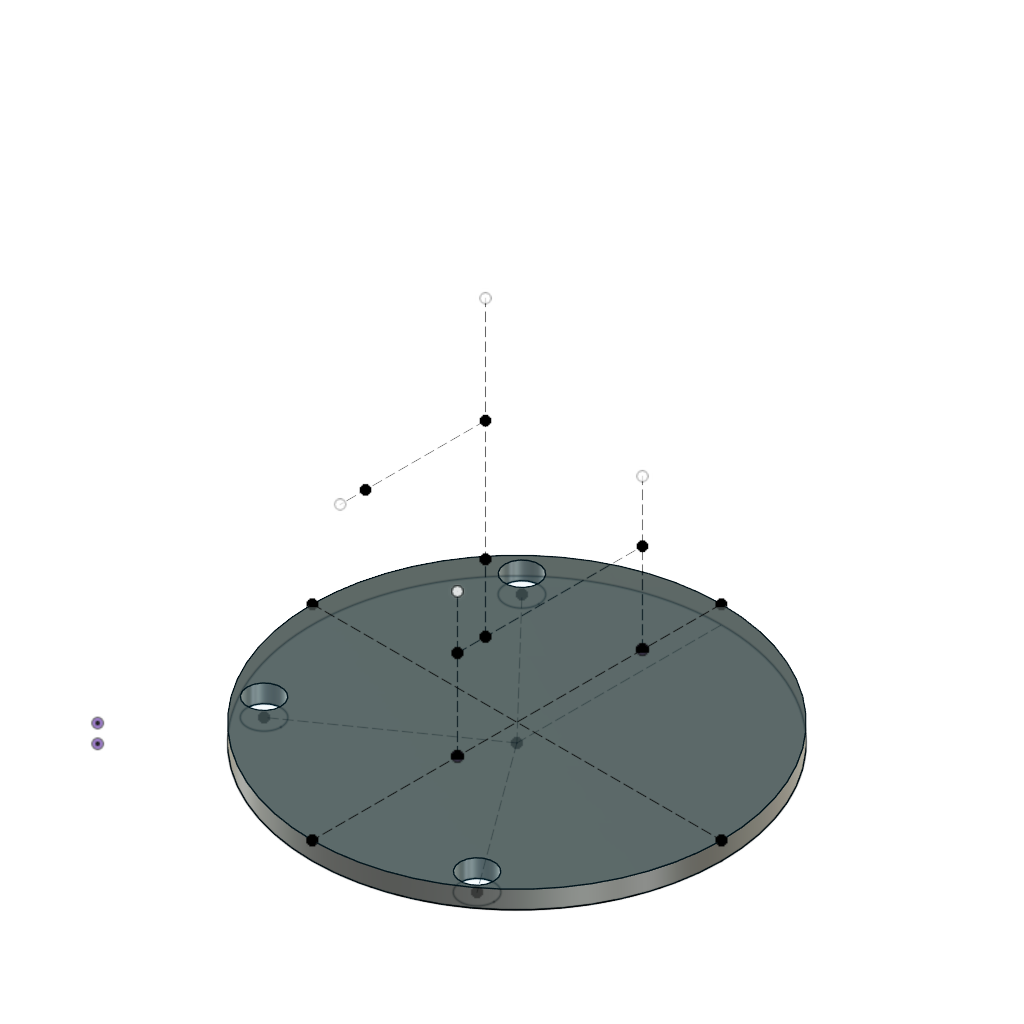
ZSB (Autodesk Fusion 360 archive; units mm, degrees)
design "Adapterplatine"
Autodesk Fusion 360 part; units mm, degrees
note: some values were not read from the file. Set by a fixed rule: which face or edge a step refers to.
sketch "Skizze1" plane through (0, 0, 0) normal (0, 0, 1) x (1, 0, 0)
  circle A0 centre (18.631, 18.76) radius 18.25
  circle A1 centre (7.381, 30.46) radius 1.5
  circle A2 centre (5.381, 9.46) radius 1.5
  circle A3 centre (28.381, 5.46) radius 1.5
  line L0 (18.631, 18.76) -> (7.381, 30.46) construction
  line L1 (18.631, 18.76) -> (5.381, 9.46) construction
  line L2 (18.631, 18.76) -> (28.381, 5.46) construction
  line L3 (18.631, 18.76) -> (18.631, 37.01) construction
  dimension "d1" = 36.5
  dimension "d4" = 18.631
  dimension "d5" = 18.76
  dimension "d6" = 3
  dimension "d7" = 7.381
  dimension "d8" = 30.46
  dimension "d9" = 9.46
  dimension "d10" = 5.381
  dimension "d11" = 5.46
  dimension "d12" = 28.381
  dimension "d24" = 43.877
  dimension "d25" = 125.065
  dimension "d26" = 143.756
  dimension "d27" = 16.2312
  dimension "d28" = 16.188
  dimension "d29" = 16.491
  constraint equal A1 A2
  constraint equal A1 A3
  constraint coincident A0.centre L0.start
  constraint coincident A1.centre L0.end
  constraint coincident A2.centre L1.end
  constraint coincident A3.centre L2.end
  constraint coincident A0 L3.end
  constraint vertical L3
  measures "d1" diameter of A0
  measures "d4" horizontal distance of origin A0.centre
  measures "d5" vertical distance of origin A0.centre
  measures "d6" diameter of A1
  measures "d7" horizontal distance of origin A1.centre
  measures "d8" vertical distance of origin A1.centre
  measures "d9" vertical distance of origin A2.centre
  measures "d10" horizontal distance of origin A2.centre
  measures "d11" vertical distance of origin A3.centre
  measures "d12" horizontal distance of origin A3.centre
  measures "d24" angle of L0 L3
  measures "d25" angle of L1 L3
  measures "d26" angle of L2 L3
  measures "d27" distance of A0.centre A1.centre
  measures "d28" distance of A0.centre A2.centre
  measures "d29" distance of A0.centre A3.centre
extrude "Extrusion1" add sketch "Skizze1" along normal blind 1.6
sketch "Skizze2" plane through (0, 0, 1.6) normal (0, 0, 1) x (-1, 0, 0)
  circle A0 centre (-5.381, -9.46) radius 1.5
  circle A1 centre (-7.381, -30.46) radius 1.5
  circle A2 centre (-28.381, -5.46) radius 1.5
  circle A3 centre (-18.631, -18.76) radius 18.25
  line L0 (-18.631, -37.01) -> (-18.631, -0.51) construction
  line L1 (-0.381, -18.76) -> (-36.881, -18.76) construction
  point P0 (-18.631, -29.96)
  point P1 (-18.631, -13.46)
  dimension "d13" = 13.46
  dimension "d15" = 29.96
  constraint coincident A3 L0.start
  constraint coincident A3 L0.end
  constraint vertical L0
  constraint coincident A3 L1.start
  constraint coincident A3 L1.end
  constraint horizontal L1
  constraint coincident A3.centre L1
  constraint coincident A3.centre L0
  constraint coincident L0 P1
  constraint coincident L0 P0
  measures "d13" vertical distance of origin P1
  measures "d15" vertical distance of origin P0
ref_plane "Arbeitsebene1" through (18.631, 0, 0) normal (1, 0, 0) x (0, 1, 0)
sketch "Skizze3" plane through (18.631, 0, 0) normal (1, 0, 0) x (0, 1, 0)
  line L0 (13.46, 1.6) -> (13.46, 14.3588) construction
  line L1 (29.96, 1.6) -> (29.96, 15) construction
  line L2 (13.46, 9.6) -> (29.96, 9.6) construction
  line L3 (15.96, 9.6) -> (15.96, 35.7478) construction
  line L4 (15.96, 26.3) -> (3, 26.3) construction
  point P0 (13.46, 1.6)
  point P1 (29.96, 1.6)
  point P2 (13.46, 9.6)
  point P3 (29.96, 9.6)
  point P4 (15.96, 9.6)
  point P5 (15.96, 15.6)
  point P6 (15.96, 26.3)
  point P7 (5.26, 26.3)
  dimension "d18" = 8
  dimension "d19" = 8
  dimension "d20" = 2.5
  dimension "d21" = 6
  dimension "d22" = 10.7
  dimension "d23" = 10.7
  constraint coincident P0 L0.start
  constraint vertical L0
  constraint coincident P1 L1.start
  constraint vertical L1
  constraint coincident L0 P2
  constraint coincident L1 P3
  constraint coincident P2 L2.start
  constraint coincident P3 L2.end
  constraint coincident L2 P4
  constraint coincident P4 L3.start
  constraint perpendicular L2 L3
  constraint coincident L3 P5
  constraint coincident L3 P6
  constraint coincident P6 L4.start
  constraint perpendicular L3 L4
  constraint coincident L4 P7
  measures "d18" distance of P0 P2
  measures "d19" distance of P1 P3
  measures "d20" distance of P2 P4
  measures "d21" distance of P4 P5
  measures "d22" distance of P5 P6
  measures "d23" distance of P6 P7
equation "d19 = d18"

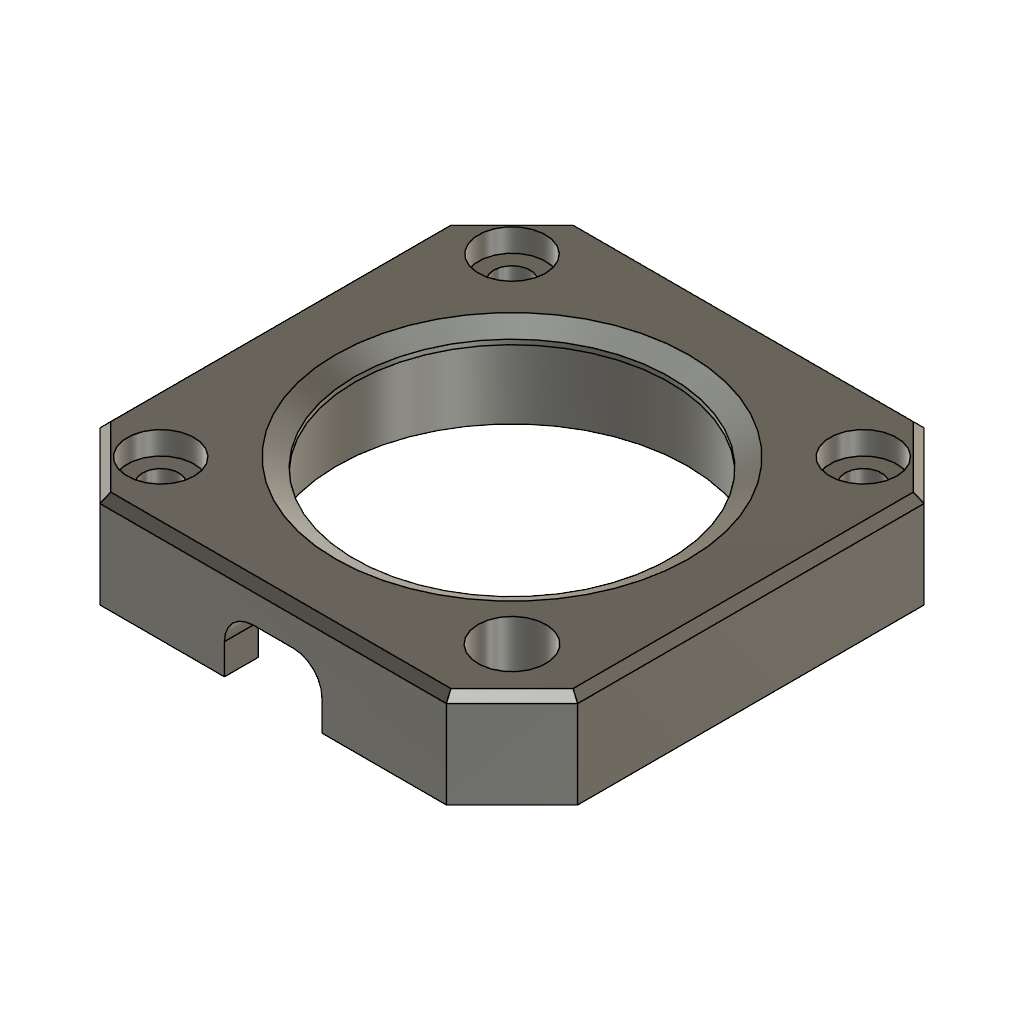
design "Frontplatte"
Autodesk Fusion 360 part; units mm, degrees
sketch "Skizze1" plane through (0, 0, 0) normal (0, 0, 1) x (1, 0, 0)
  line L0 (-50, 50) -> (0, 50)
  line L1 (0, 50) -> (0, 0)
  line L2 (0, 0) -> (-50, 0)
  line L3 (-50, 0) -> (-50, 50)
  line L4 (-50, 25) -> (0, 25) construction
  line L5 (-25, 50) -> (-25, 0) construction
  circle A0 centre (-25, 25) radius 16.5
  circle A1 centre (-8.0294, 8.0294) radius 3.55
  line L6 (-50, 50) -> (0, 0) construction
  line L7 (0, 50) -> (-50, 0) construction
  circle A2 centre (-43.3848, 43.3848) radius 1.9
  circle A3 centre (-6.6152, 43.3848) radius 1.9
  circle A4 centre (-43.3848, 6.6152) radius 1.9
  line L8 (-6.8665, 50) -> (0, 43.1335)
  line L9 (-50, 6.8665) -> (-43.1335, 0)
  line L10 (-43.1335, 50) -> (-50, 43.1335)
  line L11 (0, 6.8665) -> (-6.8665, 0)
  line L12 (-8.0294, 16.5147) -> (-16.5147, 8.0294) construction
  line L13 (-16.5147, 8.0294) -> (-8.0294, -0.4558) construction
  line L14 (-8.0294, -0.4558) -> (0.4558, 8.0294) construction
  line L15 (0.4558, 8.0294) -> (-8.0294, 16.5147) construction
  line L16 (-8.0294, 16.5147) -> (-8.0294, -0.4558) construction
  point P0 (-8.0294, 8.0294)
  point P1 (-8.0294, 8.0294)
  dimension "d3" = 33
  dimension "d4" = 7.1
  dimension "d6" = 3.8
  dimension "d7" = 26
  dimension "d8" = 26
  dimension "d9" = 26
  dimension "d42" = 50
  dimension "d43" = 50
  dimension "d44" = 61
  dimension "d45" = 61
  dimension "d46" = 12
  dimension "d47" = 12
  dimension "d54" = 6.5
  constraint horizontal L0
  constraint vertical L1
  constraint horizontal L2
  constraint vertical L3
  constraint coincident L1.end L2.start
  constraint midpoint L3 L4.start
  constraint midpoint L1 L4.end
  constraint midpoint L0 L5.start
  constraint midpoint L2 L5.end
  constraint midpoint L4 A0.centre
  constraint coincident L6 A2.centre
  constraint coincident L7 A3.centre
  constraint coincident L7 A4.centre
  constraint equal A2 A3
  constraint equal A2 A4
  constraint coincident L0 L8.start
  constraint coincident L1 L8.end
  constraint perpendicular L7 L8
  constraint coincident L3 L9.start
  constraint coincident L2 L9.end
  constraint perpendicular L7 L9
  constraint coincident L0 L10.start
  constraint coincident L3 L10.end
  constraint perpendicular L6 L10
  constraint coincident L1 L11.start
  constraint coincident L2 L11.end
  constraint symmetric L6 L8 L9
  constraint symmetric L7 L10 L11
  constraint coincident P1 P0
  constraint parallel L12 L14
  constraint vertical L16
  constraint perpendicular L12 L15
  constraint perpendicular L12 L13
  constraint midpoint L16 P1
  constraint coincident P1 L6
  measures "d3" diameter of A0
  measures "d4" diameter of A1
  measures "d6" diameter of A2
  measures "d7" distance of A0.centre A2.centre
  measures "d8" distance of A0.centre A3.centre
  measures "d9" distance of A0.centre A4.centre
  measures "d42" distance of L0.start L2.end
  measures "d43" distance of L0.start L0.end
  measures "d44" distance of L8 L9
  measures "d45" distance of L10 L11
  measures "d46" distance of L12.start L14.end
  measures "d47" distance of L12.start L12.end
  measures "d54" distance of P1 L11
extrude "Extrusion1" add sketch "Skizze1" along normal blind 3 contours L0 L1 L2 L3 L8 L9 L10 L11
chamfer "Fase1" distance 0.8 angle 45 8 edges at (-25, 0, 3) (-46.5668, 3.4332, 3) (-50, 25, 3) (-46.5668, 46.5668, 3) (-25, 50, 3) (-3.4332, 46.5668, 3) (0, 25, 3) (-3.4332, 3.4332, 3)
chamfer "Fase3" distance 2 distance2 1 1 edges at (-40.3834, 30.9667, 3) measured on face at (-24.589, 46.618, 3)
sketch "Skizze2" plane through (0, 0, 0) normal (0, 0, -1) x (1, 0, 0)
  circle A0 centre (-25, -25) radius 16.5
  circle A1 centre (-43.3848, -43.3848) radius 1.9
  circle A2 centre (-43.3848, -6.6152) radius 1.9
  circle A3 centre (-8.0294, -8.0294) radius 3.55
  circle A4 centre (-6.6152, -43.3848) radius 1.9
  line L0 (-50, -43.1335) -> (-43.1335, -50)
  line L1 (-43.1335, -50) -> (-6.8665, -50)
  line L2 (-6.8665, -50) -> (0, -43.1335)
  line L3 (0, -43.1335) -> (0, -6.8665)
  line L4 (0, -6.8665) -> (-6.8665, 0)
  line L5 (-6.8665, 0) -> (-43.1335, 0)
  line L6 (-43.1335, 0) -> (-50, -6.8665)
  line L7 (-50, -6.8665) -> (-50, -43.1335)
  circle A5 centre (-25, -25) radius 18.35
  line L8 (-14.75, -9.7796) -> (-17.9, -3.55)
  line L9 (-17.9, -3.55) -> (-32.1, -3.55)
  line L10 (-32.1, -3.55) -> (-35.25, -9.7796)
  line L11 (-25, -25) -> (-25, 4.0219) construction
  dimension "d18" = 36.7
  dimension "d19" = 21.45
  dimension "d20" = 20.5
  dimension "d21" = 14.2
  constraint concentric A0 A5
  constraint coincident A5 L8.start
  constraint horizontal L9
  constraint coincident A5 L10.end
  constraint coincident A0.centre A5.centre
  constraint vertical L11
  constraint symmetric L8.end L9.end L11
  constraint symmetric L8.start L10.end L11
  measures "d18" diameter of A5
  measures "d19" distance of A0.centre L9
  measures "d20" distance of L8.start L10.end
  measures "d21" distance of L8.end L9.end
extrude "Extrusion2" cut sketch "Skizze2" against normal blind 1.5 contours A5 | A5 L8 L9 L10
sketch "Skizze3" plane through (0, 0, 0) normal (0, -1, 0) x (1, 0, 0)
  line L0 (-6.8665, 2.2) -> (-43.1335, 2.2)
  line L1 (-43.1335, 2.2) -> (-43.1335, 0)
  line L2 (-43.1335, 0) -> (-6.8665, 0)
  line L3 (-6.8665, 0) -> (-6.8665, 2.2)
  line L4 (-41.5, 1.5) -> (-8.5, 1.5)
  line L5 (-41.5, 2) -> (-8.5, 2)
  line L6 (-25, 1.5) -> (-25, -10) construction
  line L7 (-22.9, -6.8) -> (-27.1, -6.8)
  line L8 (-22.9, -0.8) -> (-27.1, -0.8)
  arc A0 (-27.1, -0.8) -> (-27.1, -6.8) centre (-27.1, -3.8) ccw
  arc A1 (-22.9, -6.8) -> (-22.9, -0.8) centre (-22.9, -3.8) ccw
  line L9 (-19.9, -3.8) -> (-30.1, -3.8) construction
  line L10 (-25, -5.5) -> (-25, -2.1) construction
  line L11 (-22.9, -6.8) -> (-19.9, -6.8)
  line L12 (-19.9, -6.8) -> (-19.9, -3.8)
  line L13 (-27.1, -6.8) -> (-30.1, -6.8)
  line L14 (-30.1, -6.8) -> (-30.1, -3.8)
  line L15 (-30.1, -6.8) -> (-19.9, -6.8)
  line L16 (-19.9, -6.8) -> (-19.9, -8.8)
  line L17 (-19.9, -8.8) -> (-30.1, -8.8)
  line L18 (-30.1, -8.8) -> (-30.1, -6.8)
  point P0 (-25, -2.1)
  point P1 (-25, -5.5)
  point P2 (-25, -3.8)
  point P3 (-25, -3.8)
  dimension "d24" = 3.6
  dimension "d25" = 7
  dimension "d27" = 6
  dimension "d31" = 10.2
  dimension "d53" = 2
  constraint midpoint L4 L6.start
  constraint perpendicular L2 L6
  constraint coincident L6 P0
  constraint coincident L6 P1
  constraint horizontal L7
  constraint horizontal L8
  constraint tangent L7 A1
  constraint tangent L7 A0
  constraint tangent L8 A0
  constraint tangent L8 A1
  constraint symmetric L6 A1.centre A0.centre
  constraint coincident A1 L9.start
  constraint midpoint A0 L9.end
  constraint horizontal L9
  constraint coincident P1 L10.start
  constraint coincident P0 L10.end
  constraint midpoint L10 P3
  constraint midpoint L9 P3
  constraint coincident P3 P2
  constraint parallel L7 L11
  constraint perpendicular L7 L12
  constraint horizontal L13
  constraint perpendicular L13 L14
  constraint coincident L7.start A1.start
  constraint coincident L7.end A0.end
  constraint coincident L9.start L12.end
  constraint coincident L9.end L14.end
  constraint horizontal L15
  constraint vertical L16
  constraint horizontal L17
  constraint vertical L18
  constraint coincident L11.end L12.start
  measures "d24" distance of L6.start P0
  measures "d25" distance of L6.start P1
  measures "d27" distance of L7 L8
  measures "d31" distance of L9.start L9.end
  measures "d53" distance of L13.end L17.end
extrude "Extrusion3" add 1 faces at (-47.7677, 25.4366, 0) along direction (0, 0, -1) blind 7
extrude "Extrusion4" cut sketch "Skizze3" against normal up to surface (3.55 mm away) contours L7 L11 L13 L15 L16 L17 L18 | L7 L8 A0 A1 L15 | A1 L11 L12 L15 | A0 L13 L14 L15
sketch "Skizze4" plane through (0, 0, -7) normal (0, 0, -1) x (1, 0, 0)
  circle A0 centre (-43.3848, -43.3848) radius 1.9
  circle A1 centre (-6.6152, -43.3848) radius 1.9
  arc A2 (-35.25, -9.7796) -> (-14.75, -9.7796) centre (-25, -25) ccw
  arc A3 (-35.25, -9.7796) -> (-14.75, -9.7796) centre (-25, -25) ccw
  circle A4 centre (-8.0294, -8.0294) radius 3.55
  circle A5 centre (-8.0294, -8.0294) radius 3.55
  circle A6 centre (-43.3848, -6.6152) radius 1.9
  circle A7 centre (-8.0294, -8.0294) radius 3.5
  circle A8 centre (-8.0294, -8.0294) radius 5
  circle A9 centre (-6.6152, -43.3848) radius 1.1
  circle A10 centre (-6.6152, -43.3848) radius 3
  circle A11 centre (-43.3848, -43.3848) radius 1.1
  circle A12 centre (-43.3848, -43.3848) radius 3
  circle A13 centre (-43.3848, -6.6152) radius 1.1
  circle A14 centre (-43.3848, -6.6152) radius 3
  circle A15 centre (-43.3848, -43.3848) radius 1.9
  circle A16 centre (-6.6152, -43.3848) radius 1.9
  circle A17 centre (-43.3848, -6.6152) radius 1.9
  dimension "d49" = 6
  dimension "d50" = 10
  constraint concentric A4 A7
  constraint concentric A7 A8
  constraint concentric A1 A9
  constraint concentric A1 A10
  constraint concentric A0 A11
  constraint concentric A0 A12
  constraint concentric A6 A13
  constraint concentric A6 A14
  constraint equal A12 A14
  constraint equal A10 A12
  measures "d49" diameter of A14
  measures "d50" diameter of A8
extrude "Extrusion5" cut sketch "Skizze4" against normal blind 4 contours A10 | A12 | A14
extrude "Extrusion6" cut sketch "Skizze4" against normal blind 3 contours A8
sketch "Skizze5" plane through (0, 0, 3) normal (0, 0, 1) x (-1, 0, 0)
  line L0 (7.1979, -49.2) -> (42.8021, -49.2)
  line L1 (42.8021, -49.2) -> (49.2, -42.8021)
  line L2 (49.2, -42.8021) -> (49.2, -7.1979)
  line L3 (49.2, -7.1979) -> (42.8021, -0.8)
  line L4 (42.8021, -0.8) -> (7.1979, -0.8)
  line L5 (7.1979, -0.8) -> (0.8, -7.1979)
  line L6 (0.8, -7.1979) -> (0.8, -42.8021)
  line L7 (0.8, -42.8021) -> (7.1979, -49.2)
  circle A0 centre (43.3848, -43.3848) radius 1.9
  circle A1 centre (43.3848, -6.6152) radius 1.9
  circle A2 centre (6.6152, -43.3848) radius 1.9
  circle A3 centre (8.0294, -8.0294) radius 3.55
  circle A4 centre (25, -25) radius 18.5
  circle A5 centre (6.6152, -43.3848) radius 1.9
  circle A6 centre (6.6152, -43.3848) radius 1.9
  circle A7 centre (43.3848, -43.3848) radius 1.9
  circle A8 centre (43.3848, -43.3848) radius 1.9
  circle A9 centre (43.3848, -6.6152) radius 1.9
  circle A10 centre (43.3848, -6.6152) radius 1.9
  circle A11 centre (43.3848, -43.3848) radius 3.5
  circle A12 centre (43.3848, -6.6152) radius 3.5
  circle A13 centre (6.6152, -43.3848) radius 3.5
  dimension "d55" = 7
  constraint concentric A7 A11
  constraint concentric A9 A12
  constraint concentric A5 A13
  constraint equal A11 A13
  constraint equal A11 A12
  measures "d55" diameter of A11
extrude "Extrusion7" cut sketch "Skizze5" against normal blind 2.4 contours A11 | A12 | A13
sketch "Skizze6" plane through (0, 0, -7) normal (0, 0, -1) x (1, 0, 0)
  circle A0 centre (-8.0294, -8.0294) radius 5
  line L0 (-30.1, -3.55) -> (-30.1, 0)
  line L1 (-30.1, 0) -> (-43.1335, 0)
  line L2 (-43.1335, 0) -> (-50, -6.8665)
  line L3 (-50, -6.8665) -> (-50, -43.1335)
  line L4 (-50, -43.1335) -> (-43.1335, -50)
  line L5 (-43.1335, -50) -> (-6.8665, -50)
  line L6 (-6.8665, -50) -> (0, -43.1335)
  line L7 (0, -43.1335) -> (0, -6.8665)
  line L8 (0, -6.8665) -> (-6.8665, 0)
  line L9 (-6.8665, 0) -> (-19.9, 0)
  line L10 (-19.9, 0) -> (-19.9, -3.55)
  line L11 (-19.9, -3.55) -> (-17.9, -3.55)
  line L12 (-17.9, -3.55) -> (-14.75, -9.7796)
  arc A1 (-35.25, -9.7796) -> (-14.75, -9.7796) centre (-25, -25) ccw
  line L13 (-35.25, -9.7796) -> (-32.1, -3.55)
  line L14 (-32.1, -3.55) -> (-30.1, -3.55)
  circle A2 centre (-6.6152, -43.3848) radius 3
  circle A3 centre (-43.3848, -43.3848) radius 3
  circle A4 centre (-43.3848, -6.6152) radius 3
  circle A5 centre (-6.6152, -43.3848) radius 3
  circle A6 centre (-43.3848, -43.3848) radius 3
  circle A7 centre (-43.3848, -6.6152) radius 3
  circle A8 centre (-8.0294, -8.0294) radius 5
  circle A9 centre (-25, -25) radius 19.5
  dimension "d58" = 39
  constraint concentric A2 A5
  constraint concentric A3 A6
  constraint concentric A4 A7
  constraint concentric A0 A8
  constraint concentric A1 A9
  measures "d58" diameter of A9
equation "d8 = d7"
equation "d9 = d7"
equation "d54 = 6.85 mm - 0.35 mm"

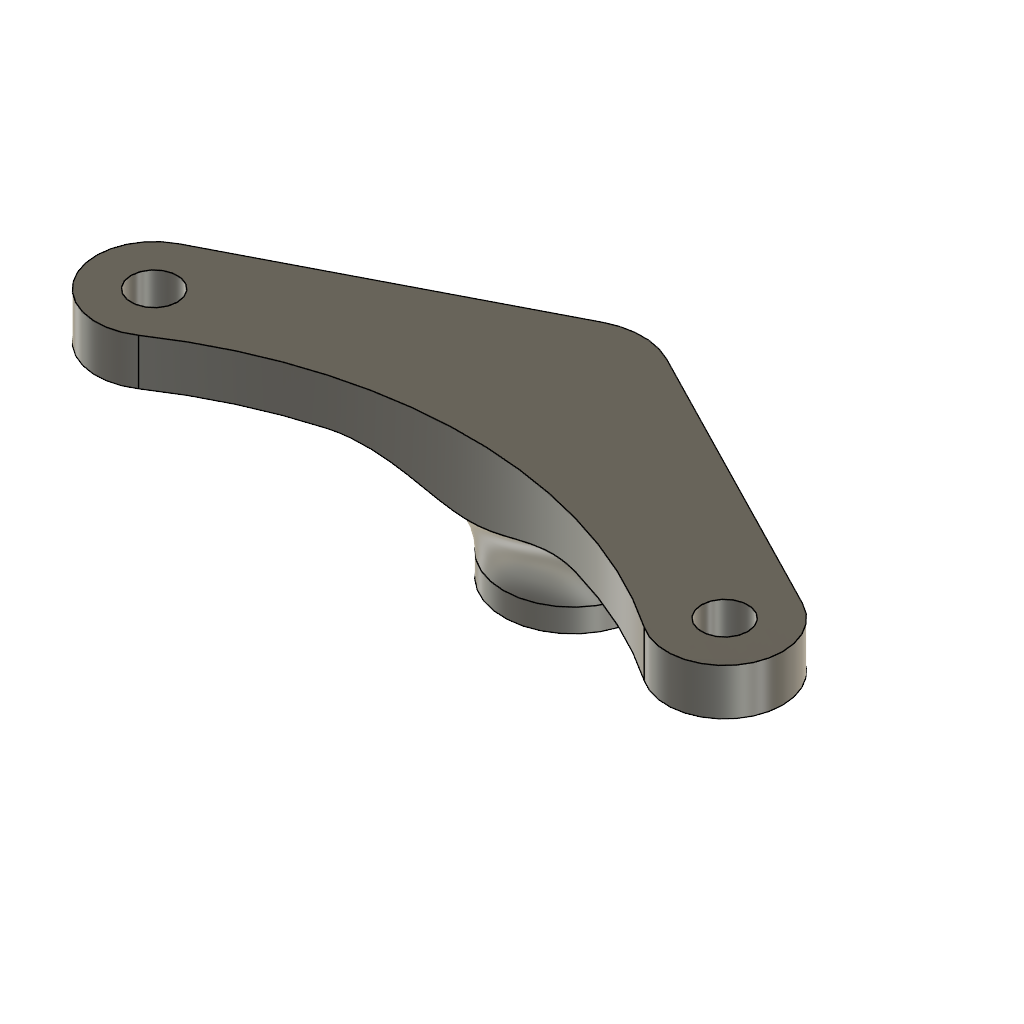
design "Haltebrücke"
Autodesk Fusion 360 part; units mm, degrees
sketch "Skizze1" plane through (0, 0, 0) normal (0, 0, 1) x (1, 0, 0)
  circle A0 centre (0, 0) radius 22 construction
  circle A1 centre (-12.3022, 18.2388) radius 1
  circle A2 centre (12.3022, 18.2388) radius 1
  line L0 (0, 0) -> (0, 38.9459) construction
  line L1 (0, 0) -> (-12.3022, 18.2388) construction
  line L2 (0, 0) -> (12.3022, 18.2388) construction
  circle A3 centre (-12.3022, 18.2388) radius 2.5
  circle A4 centre (12.3022, 18.2388) radius 2.5
  circle A5 centre (0, 24) radius 3
  line L3 (-1.3714, 26.6682) -> (-13.4451, 20.4623)
  line L4 (13.4451, 20.4623) -> (1.3714, 26.6682)
  arc A6 (10.9043, 16.1662) -> (-10.9043, 16.1662) centre (0, 0) ccw construction
  arc A7 (10.9043, 16.1662) -> (-10.9043, 16.1662) centre (0, 0) ccw
  point P0 (0, 24)
  dimension "d3" = 2
  dimension "d5" = 68
  dimension "d6" = 5
  dimension "d9" = 24
  dimension "d10" = 6
  dimension "d15" = 44
  dimension "d16" = 19.5
  constraint coincident A0.centre L0.start
  constraint coincident A0 A1.centre
  constraint coincident A0 A2.centre
  constraint vertical L0
  constraint coincident A1.centre L1.end
  constraint coincident A2.centre L2.end
  constraint symmetric A1.centre A2.centre L0
  constraint concentric A1 A3
  constraint concentric A2 A4
  constraint equal A1 A2
  constraint equal A3 A4
  constraint coincident L0 P0
  constraint coincident P0 A5.centre
  constraint coincident A5 L3.start
  constraint coincident A3 L3.end
  constraint coincident A4 L4.start
  constraint coincident A5 L4.end
  constraint tangent A5 L4
  constraint tangent A5 L3
  constraint tangent A3 L3
  constraint tangent A4 L4
  constraint concentric A0 A7
  constraint coincident L1 A6.end
  constraint coincident L2 A6.start
  constraint tangent A3 A6
  measures "d3" diameter of A1
  measures "d5" angle of L1 L2
  measures "d6" diameter of A3
  measures "d9" distance of A0.centre P0
  measures "d10" diameter of A5
  measures "d15" diameter of A0
  measures "d16" radius of A7
extrude "Extrusion1" add sketch "Skizze1" along normal blind 2
extrude "Extrusion2" add sketch "Skizze1" against normal blind 5.5 contours A5
fillet "Abrundung1" radius 4.5 1 edges at (0, 21, 0)

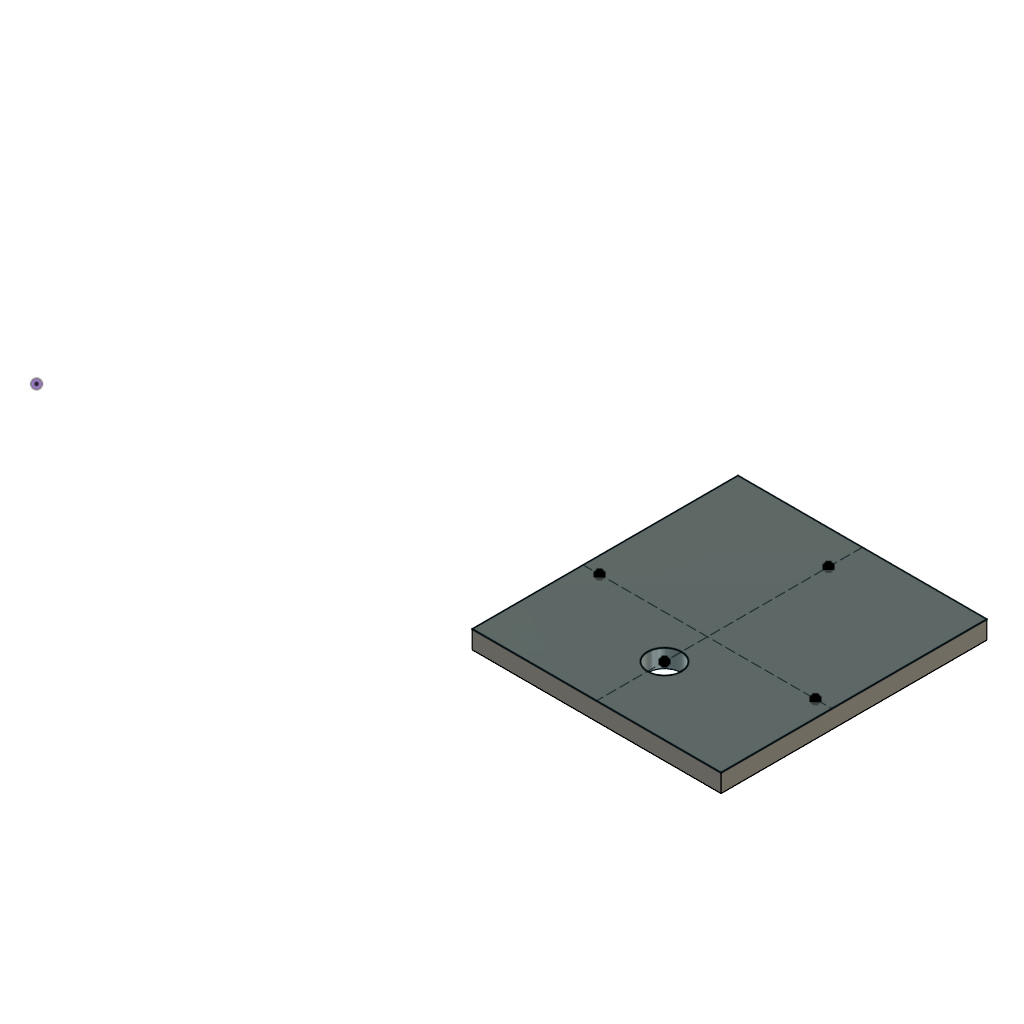
design "Adapter"
Autodesk Fusion 360 part; units mm, degrees
sketch "Skizze1" plane through (0, 0, 0) normal (0, 0, 1) x (1, 0, 0)
  line L0 (38, 23.99) -> (60, 23.99)
  line L1 (60, 23.99) -> (60, 0.49)
  line L2 (60, 0.49) -> (38, 0.49)
  line L3 (38, 0.49) -> (38, 23.99)
  circle A0 centre (49, 6.49) radius 1.5
  line L4 (49, 23.99) -> (49, 0.49) construction
  line L5 (38, 10.29) -> (60, 10.29) construction
  point P0 (39.46, 10.29)
  point P1 (58.54, 10.29)
  point P2 (49, 20.99)
  dimension "d1" = 38
  dimension "d2" = 60
  dimension "d3" = 0.49
  dimension "d4" = 23.99
  dimension "d5" = 3
  dimension "d7" = 6.49
  dimension "d8" = 10.29
  dimension "d9" = 39.46
  dimension "d10" = 58.54
  dimension "d11" = 20.99
  constraint horizontal L0
  constraint vertical L1
  constraint horizontal L2
  constraint vertical L3
  constraint midpoint L0 L4.start
  constraint midpoint L2 L4.end
  constraint coincident L3 L5.start
  constraint coincident L1 L5.end
  constraint perpendicular L1 L5
  constraint coincident A0.centre L4
  constraint coincident L5 P0
  constraint coincident L5 P1
  constraint coincident L4 P2
  measures "d1" horizontal distance of origin L2.end
  measures "d2" horizontal distance of origin L1.end
  measures "d3" vertical distance of origin L2.end
  measures "d4" vertical distance of origin L0.start
  measures "d5" diameter of A0
  measures "d7" vertical distance of origin A0.centre
  measures "d8" vertical distance of origin L5.start
  measures "d9" horizontal distance of origin P0
  measures "d10" horizontal distance of origin P1
  measures "d11" vertical distance of origin P2
extrude "Extrusion1" add sketch "Skizze1" against normal blind 1.6

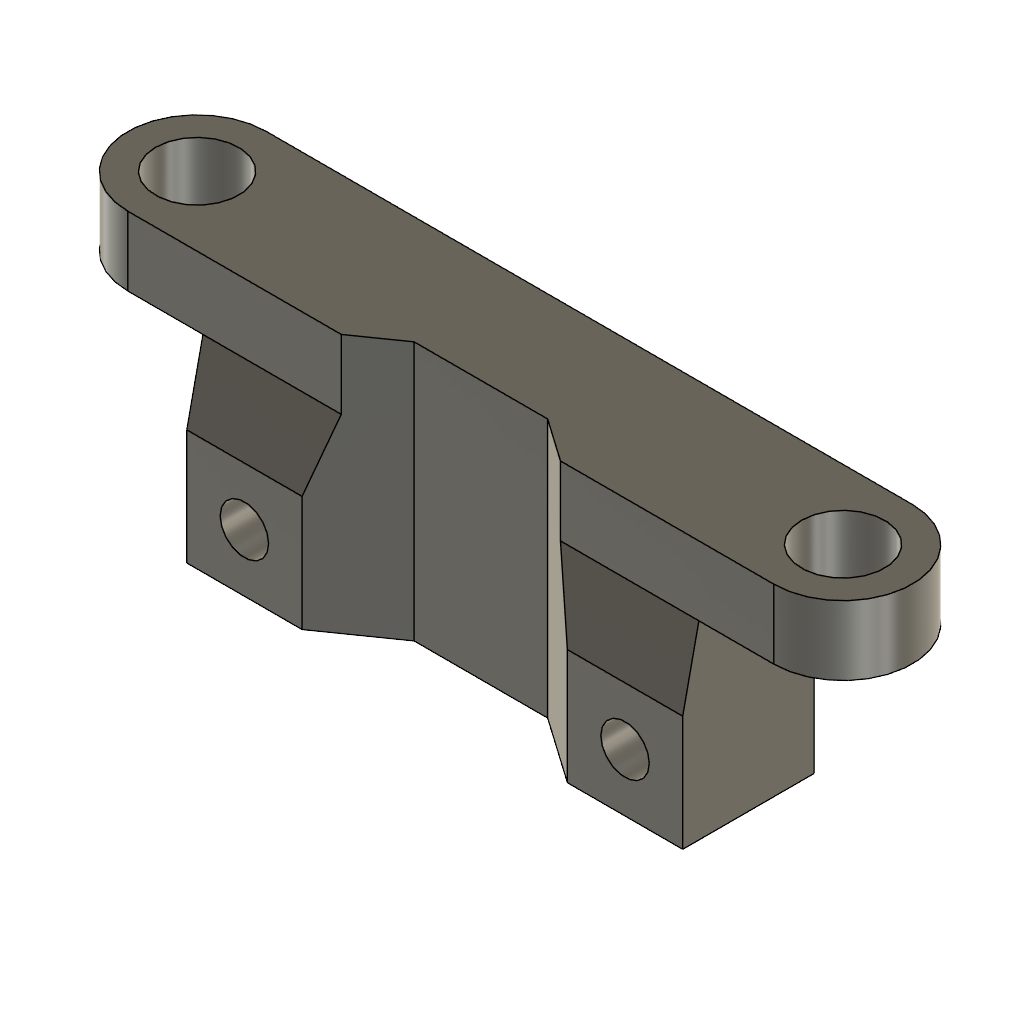
design "USB Halter"
Autodesk Fusion 360 part; units mm, degrees
sketch "Skizze1" plane through (0, 0, 0) normal (0, 0, 1) x (1, 0, 0)
  circle A0 centre (0, 0) radius 1.8
  circle A1 centre (-28, 0) radius 1.8
  line L0 (-28, 0) -> (0, 0) construction
  line L1 (-28, 3) -> (0, 3)
  line L2 (-28, -3) -> (0, -3)
  arc A2 (-28, 3) -> (-28, -3) centre (-28, 0) ccw
  arc A3 (0, -3) -> (0, 3) centre (0, 0) ccw
  dimension "d1" = 3.6
  dimension "d2" = 28
  dimension "d3" = 6
  constraint coincident A0.centre L0.end
  constraint coincident A1.centre L0.start
  constraint horizontal L0
  constraint equal A0 A1
  constraint concentric A1 A2
  constraint equal A2 A3
  constraint horizontal L1
  constraint parallel L0 L2
  constraint tangent L1 A3
  constraint tangent L2 A3
  measures "d1" diameter of A1
  measures "d2" distance of A0.centre A1.centre
  measures "d3" diameter of A2
extrude "Extrusion1" add sketch "Skizze1" along normal blind 3
sketch "Skizze2" plane through (0, 0, 0) normal (0, 0, 1) x (-1, 0, 0)
  circle A0 centre (0, 0) radius 1.8
  circle A1 centre (28, 0) radius 1.8
  arc A2 (28, -3) -> (28, 3) centre (28, 0) ccw
  line L0 (28, 3) -> (0, 3)
  arc A3 (0, 3) -> (0, -3) centre (0, 0) ccw
  line L1 (0, -3) -> (28, -3)
  line L2 (24.75, -3) -> (3.25, -3)
  line L3 (3.25, -3) -> (3.25, 3.7)
  line L4 (3.25, 3.7) -> (24.75, 3.7)
  line L5 (24.75, 3.7) -> (24.75, -3)
  circle A4 centre (0, 0) radius 1.8
  circle A5 centre (28, 0) radius 1.8
  arc A6 (28, -3) -> (28, 3) centre (28, 0) ccw
  line L6 (28, -3) -> (0, -3)
  arc A7 (0, 3) -> (0, -3) centre (0, 0) ccw
  line L7 (0, 3) -> (28, 3)
  line L8 (28, 0) -> (0, 0) construction
  line L9 (14, 0) -> (14, 18.5057) construction
  dimension "d9" = 0.7
  dimension "d10" = 21.5
  constraint horizontal L2
  constraint vertical L3
  constraint horizontal L4
  constraint vertical L5
  constraint coincident L1 L2.start
  constraint coincident A1.centre A2.centre
  constraint coincident A0.centre A3.centre
  constraint midpoint L8 L9.start
  constraint perpendicular L8 L9
  constraint symmetric L3 L5 L9
  measures "d9" distance of L0 L4
  measures "d10" distance of L3.end L4.end
extrude "Extrusion2" add sketch "Skizze2" against normal blind 8.23 contours L0 L1 L2 L3 L5 L6 L7 | L0 L3 L4 L5 L7
sketch "Skizze3" plane through (0, 3, 0) normal (0, 1, 0) x (-1, 0, 0)
  line L0 (24.75, 0) -> (28, 0)
  line L1 (28, 0) -> (28, 3)
  line L2 (28, 3) -> (0, 3)
  line L3 (0, 3) -> (0, 0)
  line L4 (0, 0) -> (3.25, 0)
  line L5 (3.25, 0) -> (3.25, -8.23)
  line L6 (3.25, -8.23) -> (24.75, -8.23)
  line L7 (24.75, -8.23) -> (24.75, 0)
  circle A0 centre (22.25, -5.73) radius 1.05
  circle A1 centre (5.75, -5.73) radius 1.05
  line L8 (24.75, -5.73) -> (3.25, -5.73) construction
  dimension "d11" = 2.1
  dimension "d13" = 2.5
  dimension "d14" = 2.5
  dimension "d15" = 2.5
  constraint coincident L7 L8.start
  constraint coincident L5 L8.end
  constraint perpendicular L5 L8
  constraint coincident A1.centre L8
  constraint coincident A0.centre L8
  constraint equal A0 A1
  measures "d11" diameter of A0
  measures "d13" distance of L7 A0.centre
  measures "d14" distance of L5 A1.centre
  measures "d15" distance of L6 L8
extrude "Extrusion3" cut sketch "Skizze3" against normal up to surface (6.7 mm away) contours A0 | A1
chamfer "Fase1" distance 1 angle 45 3 edges at (-24.75, 3, -4.115) (-14, 3, -8.23) (-3.25, 3, -4.115)
sketch "Skizze4" plane through (-24.75, 0, 0) normal (-1, 0, 0) x (0, -1, 0)
  line L0 (-2, 0) -> (-2, -8.23)
  line L1 (-2, -8.23) -> (3.7, -8.23)
  line L2 (3.7, -8.23) -> (3.7, 0)
  line L3 (3.7, 0) -> (3, 0)
  line L4 (3, 0) -> (-2, 0)
  line L5 (3.7, -4.68) -> (3.7, -6.78)
  line L6 (3.7, -4.68) -> (3.7, -6.78)
  line L7 (3.7, 0) -> (3.7, -8.23)
  line L8 (3.7, -8.23) -> (3.7, 0)
  line L9 (3, 0) -> (3, 3)
  line L10 (3, 3) -> (3, 0)
  line L11 (3, 0) -> (3.7, 0)
  line L12 (3.7, 0) -> (3, 0)
  line L13 (3.7, -3.23) -> (3.7, 0)
  line L14 (3, 0) -> (3.7, -3.23)
  dimension "d29" = 5
  constraint coincident L8 L13.start
  constraint coincident L2.end L3.start
  constraint coincident L3.end L4.start
  measures "d29" distance of L1.end L13.start
extrude "Extrusion4" cut sketch "Skizze4" against normal up to surface (21.5 mm away) contours L2 L3 L7 L8 L11 L12 L13 L14
sketch "Skizze5" plane through (0, 0, -8.23) normal (0, 0, -1) x (1, 0, 0)
  line L0 (-24.75, -2) -> (-3.25, -2)
  line L1 (-3.25, -2) -> (-3.25, 3.7)
  line L2 (-3.25, 3.7) -> (-24.75, 3.7)
  line L3 (-24.75, 3.7) -> (-24.75, -2)
  line L4 (-19.75, 3.7) -> (-16.8937, 1.7)
  line L5 (-16.8937, 1.7) -> (-11.1063, 1.7)
  line L6 (-11.1063, 1.7) -> (-8.25, 3.7)
  line L7 (-14, 3.7) -> (-14, -2) construction
  line L8 (-19.75, 3.7) -> (-8.25, 3.7)
  dimension "d22" = 5
  dimension "d24" = 2
  dimension "d25" = 35
  constraint coincident L2 L4.start
  constraint horizontal L5
  constraint coincident L2 L6.end
  constraint midpoint L2 L7.start
  constraint midpoint L0 L7.end
  constraint symmetric L4.end L5.end L7
  constraint symmetric L4.start L6.end L7
  measures "d22" distance of L2.end L4.start
  measures "d24" distance of L5 L8
  measures "d25" angle of L4 L8
extrude "Extrusion5" cut sketch "Skizze5" against normal up to surface (11.23 mm away) contours L2 L4 L5 L6 L8
equation "d7 = -6.73 mm - 1.5 mm"
equation "d13 = 1 mm + 1.5 mm"
equation "d14 = 1 mm + 1.5 mm"
equation "d15 = 1 mm + 1.5 mm"
equation "d22 = 1 mm + 3 mm + 1 mm"
equation "d29 = 1 mm + 3 mm + 1 mm"

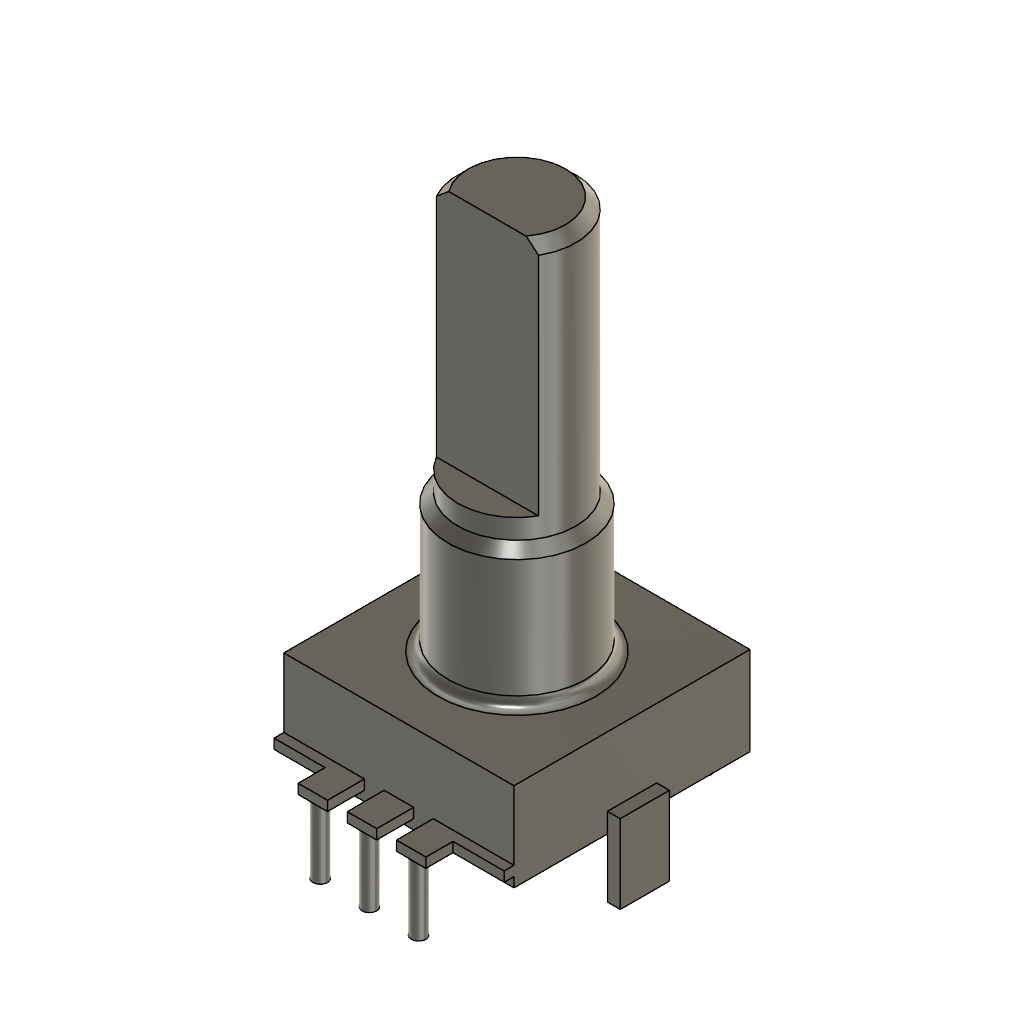
design "EC11E single rotary"
Autodesk Fusion 360 part; units mm, degrees
sketch "Skizze1" plane through (0, 0, 0) normal (0, 0, 1) x (1, 0, 0)
  line L0 (0, 0) -> (-11.7, 0)
  line L1 (-11.7, 0) -> (-11.7, 12)
  line L2 (-11.7, 12) -> (0, 12)
  line L3 (0, 12) -> (0, 0)
  dimension "d1" = 11.7
  dimension "d2" = 12
  constraint horizontal L0
  constraint vertical L1
  constraint horizontal L2
  constraint vertical L3
  constraint coincident L0.start L3.end
  measures "d1" distance of L1.end L2.end
  measures "d2" distance of L0.end L1.end
extrude "Extrusion1" add sketch "Skizze1" along normal blind 4.5
ref_plane "Arbeitsebene1" through (0, 0, 0.5) normal (0, 0, 1) x (1, 0, 0)
sketch "Skizze2" plane through (0, 0, 0.5) normal (0, 0, 1) x (1, 0, 0)
  line L0 (0, 12) -> (-11.7, 12)
  line L1 (-11.7, 12) -> (-11.7, 0)
  line L2 (-11.7, 0) -> (0, 0)
  line L3 (0, 0) -> (0, 12)
  line L4 (-8.35, 12) -> (-8.35, 19) construction
  line L5 (-3.35, 12) -> (-3.35, 19) construction
  line L6 (-8.35, 0) -> (-8.35, -5) construction
  line L7 (-5.85, 0) -> (-5.85, -5) construction
  line L8 (-3.35, 0) -> (-3.35, -5) construction
  line L9 (-7.6, 12) -> (-9.1, 12)
  line L10 (-9.1, 12) -> (-9.1, 13.375)
  line L11 (-9.1, 13.375) -> (-7.6, 13.375)
  line L12 (-7.6, 13.375) -> (-7.6, 12)
  line L13 (-2.6, 12) -> (-4.1, 12)
  line L14 (-4.1, 12) -> (-4.1, 13.375)
  line L15 (-4.1, 13.375) -> (-2.6, 13.375)
  line L16 (-2.6, 13.375) -> (-2.6, 12)
  line L17 (-2.6, 0) -> (-4.1, 0)
  line L18 (-4.1, 0) -> (-4.1, -1.875)
  line L19 (-4.1, -1.875) -> (-2.6, -1.875)
  line L20 (-2.6, -1.875) -> (-2.6, 0)
  line L21 (-6.6, 0) -> (-5.1, 0)
  line L22 (-5.1, 0) -> (-5.1, -1.875)
  line L23 (-5.1, -1.875) -> (-6.6, -1.875)
  line L24 (-6.6, -1.875) -> (-6.6, 0)
  line L25 (-9.1, 0) -> (-7.6, 0)
  line L26 (-7.6, 0) -> (-7.6, -1.875)
  line L27 (-7.6, -1.875) -> (-9.1, -1.875)
  line L28 (-9.1, -1.875) -> (-9.1, 0)
  line L29 (-9.1, 0) -> (-11.7, 0)
  line L30 (-11.7, 0) -> (-11.7, -0.5)
  line L31 (-11.7, -0.5) -> (-9.1, -0.5)
  line L32 (-9.1, -0.5) -> (-9.1, 0)
  line L33 (-2.6, 0) -> (0, 0)
  line L34 (0, 0) -> (0, -0.5)
  line L35 (0, -0.5) -> (-2.6, -0.5)
  line L36 (-2.6, -0.5) -> (-2.6, 0)
  circle A0 centre (-8.35, 13) radius 0.375
  circle A1 centre (-3.35, 13) radius 0.375
  circle A2 centre (-8.35, -1.5) radius 0.375
  circle A3 centre (-5.85, -1.5) radius 0.375
  circle A4 centre (-3.35, -1.5) radius 0.375
  line L37 (-11.7, 6) -> (0, 6) construction
  line L38 (-11.7, 7.25) -> (-12.35, 7.25)
  line L39 (-12.35, 7.25) -> (-12.35, 4.75)
  line L40 (-12.35, 4.75) -> (-11.7, 4.75)
  line L41 (-11.7, 4.75) -> (-11.7, 7.25)
  line L42 (0, 7.25) -> (0.65, 7.25)
  line L43 (0.65, 7.25) -> (0.65, 4.75)
  line L44 (0.65, 4.75) -> (0, 4.75)
  line L45 (0, 4.75) -> (0, 7.25)
  line L46 (-11.6, 7.25) -> (-11.6, 4.75)
  line L47 (-0.1, 7.25) -> (-0.1, 4.75)
  dimension "d7" = 5
  dimension "d8" = 5
  dimension "d9" = 1.5
  dimension "d11" = 0.5
  dimension "d12" = 0.75
  dimension "d13" = 0.75
  dimension "d14" = 0.75
  dimension "d15" = 0.75
  dimension "d16" = 0.75
  dimension "d17" = 7
  dimension "d18" = 7
  dimension "d19" = 7.5
  dimension "d20" = 7.5
  dimension "d21" = 7.5
  dimension "d26" = 0.75
  dimension "d27" = 0.75
  dimension "d28" = 13
  dimension "d46" = 2.5
  constraint coincident L0 L4.start
  constraint perpendicular L0 L4
  constraint coincident L0 L5.start
  constraint perpendicular L0 L5
  constraint coincident L2 L6.start
  constraint perpendicular L2 L6
  constraint midpoint L2 L7.start
  constraint perpendicular L2 L7
  constraint coincident L2 L8.start
  constraint perpendicular L2 L8
  constraint horizontal L9
  constraint vertical L10
  constraint horizontal L11
  constraint vertical L12
  constraint coincident L0 L9.start
  constraint horizontal L13
  constraint vertical L14
  constraint horizontal L15
  constraint vertical L16
  constraint coincident L0 L13.start
  constraint horizontal L17
  constraint vertical L18
  constraint horizontal L19
  constraint vertical L20
  constraint coincident L2 L17.start
  constraint horizontal L21
  constraint vertical L22
  constraint horizontal L23
  constraint vertical L24
  constraint coincident L2 L21.start
  constraint horizontal L25
  constraint vertical L26
  constraint horizontal L27
  constraint vertical L28
  constraint coincident L2 L25.start
  constraint symmetric L6.end L7 L8.end
  constraint symmetric L4.end L5.end L7
  constraint symmetric L4 L10 L12
  constraint symmetric L5 L14 L16
  constraint symmetric L7 L22 L24
  constraint equal L10 L14
  constraint equal L11 L15
  constraint equal L11 L27
  constraint equal L23 L27
  constraint equal L19 L23
  constraint horizontal L29
  constraint vertical L30
  constraint horizontal L31
  constraint vertical L32
  constraint horizontal L33
  constraint vertical L34
  constraint horizontal L35
  constraint vertical L36
  constraint equal L30 L34
  constraint coincident L1.end L2.start
  constraint coincident L4 A0.centre
  constraint coincident L5 A1.centre
  constraint coincident L6 A2.centre
  constraint coincident L7 A3.centre
  constraint coincident L8 A4.centre
  constraint midpoint L1 L37.start
  constraint midpoint L3 L37.end
  constraint tangent L11 A0
  constraint tangent L27 A2
  constraint tangent L23 A3
  constraint tangent L19 A4
  constraint horizontal L38
  constraint vertical L39
  constraint horizontal L40
  constraint vertical L41
  constraint coincident L1 L38.start
  constraint horizontal L42
  constraint vertical L43
  constraint horizontal L44
  constraint vertical L45
  constraint coincident L3 L42.start
  constraint symmetric L37 L38 L40
  constraint symmetric L37 L42 L44
  constraint equal L38 L42
  constraint equal L39 L43
  constraint coincident L38 L46.start
  constraint coincident L40 L46.end
  constraint perpendicular L40 L46
  constraint coincident L42 L47.start
  constraint coincident L44 L47.end
  constraint perpendicular L44 L47
  measures "d7" distance of L4 L5
  measures "d8" distance of L6 L8
  measures "d9" distance of L10.end L11.end
  measures "d11" distance of L1.end L30.end
  measures "d12" diameter of A0
  measures "d13" diameter of A1
  measures "d14" diameter of A2
  measures "d15" diameter of A3
  measures "d16" diameter of A4
  measures "d17" distance of A0.centre L37
  measures "d18" distance of A1.centre L37
  measures "d19" distance of A2.centre L37
  measures "d20" distance of A3.centre L37
  measures "d21" distance of A4.centre L37
  measures "d26" distance of L39 L46
  measures "d27" distance of L43 L47
  measures "d28" distance of L39 L43
  measures "d46" distance of L38.end L39.end
extrude "Extrusion2" add sketch "Skizze2" along normal blind 0.5 contours A1 | L0 L13 L14 L15 L16 | L3 L42 L43 L44 L45 | A0 | L0 L9 L10 L11 L12 | L2 L20 L33 L34 L35 L36 | A4 | L2 L17 L18 L19 L20 L36 | L1 L38 L39 L40 L41 | A3 | L2 L21 L22 L23 L24 | L2 L28 L29 L30 L31 L32 | A2 | L2 L25 L26 L27 L28 L32
extrude "Extrusion3" add sketch "Skizze2" against normal blind 3.5 contours A1 | L3 L42 L43 L44 L45 | A0 | A4 | L1 L38 L39 L40 L41 | A3 | A2
ref_plane "Arbeitsebene2" through (0, 6, 0) normal (0, 1, 0) x (0, 0, 1)
sketch "Skizze3" plane through (0, 6, 0) normal (0, 1, 0) x (1, 0, 0)
  line L0 (-4.1, -1) -> (0, -1)
  line L1 (0, -1) -> (0, -4.5)
  line L2 (0, -4.5) -> (-11.7, -4.5)
  line L3 (-11.7, -4.5) -> (-11.7, -1)
  line L4 (-11.7, -1) -> (-7.6, -1)
  line L5 (-7.6, -1) -> (-7.6, -0.5)
  line L6 (-7.6, -0.5) -> (-11.7, -0.5)
  line L7 (-11.7, -0.5) -> (-11.7, 0)
  line L8 (-11.7, 0) -> (0, 0)
  line L9 (0, 0) -> (0, -0.5)
  line L10 (0, -0.5) -> (-4.1, -0.5)
  line L11 (-4.1, -0.5) -> (-4.1, -1)
  line L12 (-5.1, -1) -> (-5.1, -0.5)
  line L13 (-5.1, -0.5) -> (-6.6, -0.5)
  line L14 (-6.6, -0.5) -> (-6.6, -1)
  line L15 (-6.6, -1) -> (-5.1, -1)
  line L16 (-5.85, -4.5) -> (-5.85, -18.5)
  line L17 (-5.85, -4.5) -> (-1.85, -4.5)
  line L18 (-2.35, -5) -> (-2.35, -11)
  arc A0 (-1.85, -4.5) -> (-2.35, -5) centre (-1.85, -5) ccw
  line L19 (-2.35, -11) -> (-2.85, -11.5)
  line L20 (-2.85, -11.5) -> (-2.85, -23.9697)
  line L21 (-2.85, -23.9697) -> (-3.3803, -24.5)
  line L22 (-3.3803, -24.5) -> (-5.85, -24.5)
  line L23 (-5.85, -24.5) -> (-5.85, -4.5)
  dimension "d31" = 1
  dimension "d32" = 7
  dimension "d33" = 6
  dimension "d34" = 135
  dimension "d35" = 135
  dimension "d36" = 7
  dimension "d40" = 0.75
  dimension "d41" = 20
  constraint midpoint L2 L16.start
  constraint perpendicular L2 L16
  constraint tangent L17 A0
  constraint vertical L18
  constraint tangent L18 A0
  constraint parallel L18 L20
  constraint coincident L16 L22.end
  constraint perpendicular L16 L22
  constraint horizontal L17
  measures "d31" diameter of A0
  measures "d34" angle of L18 L19
  measures "d35" angle of L20 L21
  measures "d36" distance of L17 L19.end
  measures "d40" distance of L20.end L21.end
  measures "d41" distance of L2 L22
revolve "Drehen1" add sketch "Skizze3" angle 360 about axis through (-5.85, 6, 4.5) along (0, 0, 1) contours L2 L16 L17 L18 A0 L19 L20 L21 L22 L23
sketch "Skizze4" plane through (0, 0, 24.5) normal (0, 0, 1) x (-1, 0, 0)
  circle A0 centre (5.85, -6) radius 2.4697
  circle A1 centre (5.85, -6) radius 3
  line L0 (8.4481, -4.5) -> (3.2519, -4.5)
  arc A2 (8.4481, -4.5) -> (3.2519, -4.5) centre (5.85, -6) ccw
  line L1 (5.85, -4.5) -> (5.85, -9) construction
  dimension "d43" = 4.5
  constraint coincident A1 L0.start
  constraint coincident A1 L0.end
  constraint horizontal L0
  constraint concentric A1 A2
  constraint midpoint L0 L1.start
  constraint coincident A1 L1.end
  constraint perpendicular A1 L1
  measures "d43" distance of L1.start L1.end
extrude "Extrusion4" cut sketch "Skizze4" against normal blind 12 contours A0 L0 | A0 A1 L0 A2 picked at (5.6769, -4.1952)
equation "d13 = d12"
equation "d14 = d12"
equation "d15 = d12"
equation "d16 = d12"

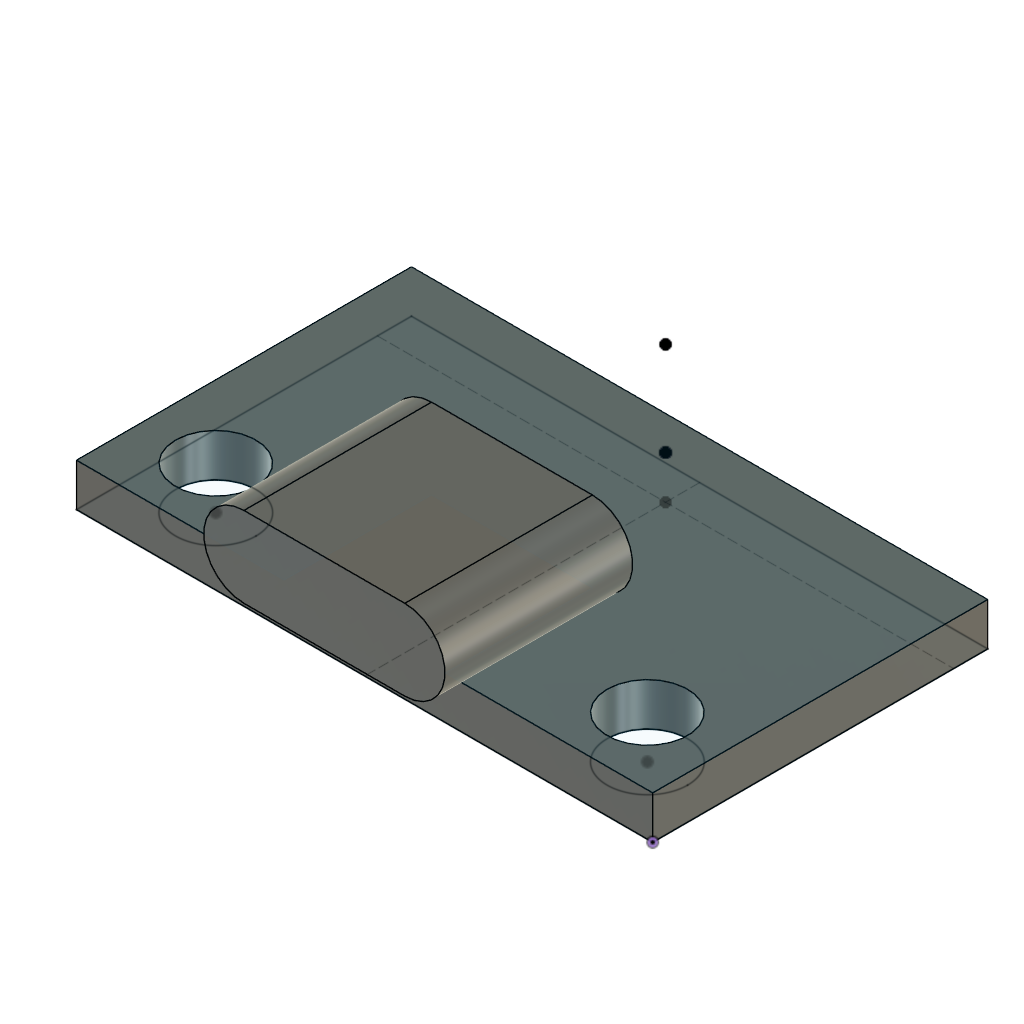
design "USB-Breakout"
Autodesk Fusion 360 part; units mm, degrees
sketch "Skizze1" plane through (0, 0, 0) normal (0, 0, 1) x (1, 0, 0)
  line L0 (0, 0) -> (-21.5, 0)
  line L1 (-21.5, 0) -> (-21.5, 12.5)
  line L2 (-21.5, 12.5) -> (0, 12.5)
  line L3 (0, 12.5) -> (0, 0)
  circle A0 centre (-18.8, 2.5) radius 1.5
  circle A1 centre (-2.7, 2.5) radius 1.5
  line L4 (-21.5, 11.23) -> (0, 11.23) construction
  line L5 (-10.75, 12.5) -> (-10.75, 0) construction
  point P0 (-10.75, 11.23)
  dimension "d1" = 21.5
  dimension "d2" = 12.5
  dimension "d3" = 3
  dimension "d4" = 2.7
  dimension "d5" = 2.7
  dimension "d6" = 2.5
  dimension "d7" = 2.5
  dimension "d8" = 1.27
  constraint horizontal L0
  constraint vertical L1
  constraint horizontal L2
  constraint vertical L3
  constraint coincident L0.start L3.end
  constraint equal A0 A1
  constraint coincident L1 L4.start
  constraint coincident L3 L4.end
  constraint perpendicular L3 L4
  constraint midpoint L2 L5.start
  constraint midpoint L0 L5.end
  constraint midpoint L4 P0
  measures "d1" distance of L1.end L2.end
  measures "d2" distance of L0.end L1.end
  measures "d3" diameter of A0
  measures "d4" distance of L1 A0.centre
  measures "d5" distance of L3 A1.centre
  measures "d6" distance of L0 A0.centre
  measures "d7" distance of L0 A1.centre
  measures "d8" distance of L2 L4
extrude "Extrusion1" add sketch "Skizze1" along normal blind 1.6
sketch "Skizze2" plane through (0, 0, 0) normal (0, -1, 0) x (1, 0, 0)
  line L0 (-21.5, 0) -> (0, 0)
  line L1 (0, 0) -> (0, 1.6)
  line L2 (0, 1.6) -> (-21.5, 1.6)
  line L3 (-21.5, 1.6) -> (-21.5, 0)
  line L4 (-10.75, 0) -> (-10.75, 13.6465) construction
  line L5 (-13.75, 4.6) -> (-7.75, 4.6)
  line L6 (-7.75, 1.6) -> (-13.75, 1.6)
  arc A0 (-13.75, 4.6) -> (-13.75, 1.6) centre (-13.75, 3.1) ccw
  arc A1 (-7.75, 1.6) -> (-7.75, 4.6) centre (-7.75, 3.1) ccw
  point P0 (-10.75, 1.6)
  dimension "d11" = 1.5
  dimension "d12" = 6
  constraint midpoint L0 L4.start
  constraint perpendicular L2 L4
  constraint tangent L5 A1
  constraint tangent L6 A0
  constraint tangent L5 A0
  constraint tangent L6 A1
  constraint equal A0 A1
  constraint symmetric L4 L5.start L5.end
  constraint midpoint L2 P0
  constraint coincident L6 P0
  measures "d11" radius of A0
  measures "d12" distance of A0.centre A1.centre
extrude "Extrusion2" add sketch "Skizze2" along normal blind 1.5 and the other way blind 5.5 contours L2 L5 L6 A0 A1
sketch "Skizze3" plane through (0, 0, 1.6) normal (0, 0, 1) x (-1, 0, 0)
  line L0 (7.75, -5.5) -> (7.75, 0)
  line L1 (7.75, 0) -> (0, 0)
  line L2 (0, 0) -> (0, -12.5)
  line L3 (0, -12.5) -> (21.5, -12.5)
  line L4 (21.5, -12.5) -> (21.5, 0)
  line L5 (21.5, 0) -> (13.75, 0)
  line L6 (13.75, 0) -> (13.75, -5.5)
  line L7 (13.75, -5.5) -> (7.75, -5.5)
  circle A0 centre (2.7, -2.5) radius 1.5
  circle A1 centre (18.8, -2.5) radius 1.5
  point P0 (10.75, -11.23)
  point P1 (10.75, -11.23)
  constraint coincident P1 P0
ref_plane "Arbeitsebene1" through (0, 0, 5.1) normal (0, 0, 1) x (1, 0, 0)
sketch "Skizze4" plane through (0, 0, 5.1) normal (0, 0, 1) x (1, 0, 0)
  point P0 (-10.75, 11.23)
  point P1 (-10.75, 11.23)
  constraint coincident P0 P1
equation "d4 = 1.2 mm + 1.5 mm"
equation "d5 = d4"
equation "d7 = d6"
equation "d8 = ( 2.54 / 2 ) * 1 mm"
equation "d12 = 9 mm - 3 mm"
equation "d15 = 7 mm - 1.5 mm"
equation "d17 = 1.6 mm + 3.5 mm"
